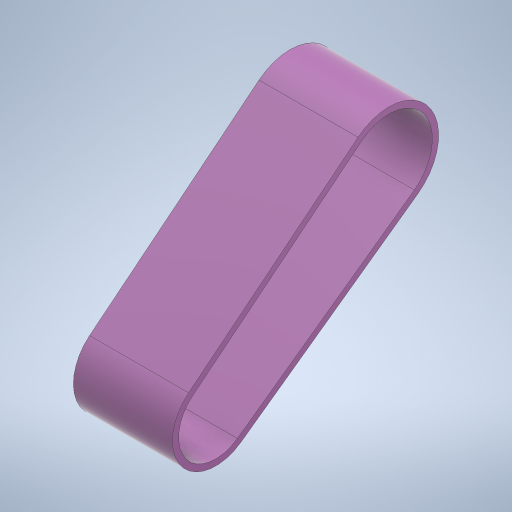
# Autodesk Inventor part: banda
Saved by Autodesk Inventor 2023 (Build 270158000, 158)
## iProperties
Created: 2022-04-04
Part Number: banda
Material: Genérico
Document SubType Name: Modeling
Designer: isaac
Density: 1 g/cm^3
Appearance: Valor por defecto
Author: isaac
Autodesk Inventor part; units mm, degrees
ref_plane "YZ Plane" through (0, 0, 0) normal (1, 0, 0) x (0, 1, 0)
ref_plane "XZ Plane" through (0, 0, 0) normal (0, 1, 0) x (-1, 0, 0)
ref_plane "XY Plane" through (0, 0, 0) normal (0, 0, 1) x (1, 0, 0)
sketch "Boceto1" plane through (0, 0, 0) normal (1, 0, 0) x (0, 1, 0)
  arc A0 (4.672, 23.7647) -> (-4.8784, 16.507) centre (0, 20) ccw
  arc A1 (15.5865, -12.0751) -> (26.7286, -3.6079) centre (21.278, -8) ccw
  line L0 (26.7286, -3.6079) -> (4.672, 23.7647)
  line L1 (-4.8784, 16.507) -> (15.5865, -12.0751)
  arc A2 (14.7734, -12.6573) -> (27.5073, -2.9805) centre (21.278, -8) ccw
  arc A3 (5.4506, 24.3921) -> (-5.6915, 15.9249) centre (0, 20) ccw
  line L2 (27.5073, -2.9805) -> (5.4506, 24.3921)
  line L3 (-5.6915, 15.9249) -> (14.7734, -12.6573)
  point P0 (0, 0)
  dimension "d2" = 6
  dimension "d3" = 7
  dimension "d4" = 8
  dimension "d5" = 20
  dimension "d6" = 3.259
  dimension "d7" = 16
  dimension "d8" = 14
  constraints: 10 point on circle, 8 end point, 7 tangent, 4 centre point, 2 coincident, 2 point on line, 1 parallel, 1 vertical alignment
  measures "d2" radius of A0
  measures "d3" radius of A1
  measures "d4" vertical distance of point (0, 0) A1.centre
  measures "d5" distance of point (0, 0) A0.centre
  measures "d6" angle of L1 L0
  measures "d7" diameter of A2
  measures "d8" diameter of A3
extrude "Extrusión1" add sketch "Boceto1" along normal blind 16
